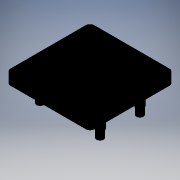
# Autodesk Inventor part: HFC5-2020-B
Saved by Autodesk Inventor 2017.3 (Build 213256000, 256)
## iProperties
Part Number: HFC5-2020-B
Material: Generic
Catalog Web Link: www.cadenas.de
Description: HFC5, HFCL5-Extrusion End Caps - HFS5 Series (Aluminum Extrusions 20, 25, 40 Square)
Vendor: MISUMI
Document SubType Name: Modeling
Designer: partserver
Manufacturer: MISUMI
Mass: 0.806307 g
Surface Area: 12.096 cm^2
Volume: 0.806307 cm^3
Density: 1 g/cm^3
Appearance: PSOLRGB-0-0-0
Category: PARTsolutions
Company: MISUMI
Title: HFC5-2020-B
Author: Cadenas PARTsolutions
Comments: Extrusion End Caps - HFS5 Series (Aluminum Extrusions 20, 25, 40 Square)
PSOL_IDENT_0: {$CADENAS_DATA\23d-libs\misumi\metric\38_al_extrusions_blackets\hfc5.prj},176 {VTYP=3D},{NB=HFC5-202
PSOL_IDENT_1: 0-B},{LINA=HFC5-2020-B},{NN=HFC5, HFCL5},{DATE=16.12.2019 05:49:00},{GEOMDATE=09.12.2019 01:53:00},{
PSOL_IDENT_2: VERSION=},{LINEID=10},{WBVAR=MAT,COLOR},{WBNUMERIC=}  {NB=HFC5-2020-B},{LINA=HFC5-2020-B},{KT=HFC5},
PSOL_IDENT_3: {PN=HFC5-2020-B},{TYPE=HFC5},{MAT=P},{MATALG='P','Polyamide','LDP','Low Density Polyethylene'},{NO=2
PSOL_IDENT_4: 020},{COLOR=B},{COL=0.00,0.00,0.00,0.00},{SHP3D=2020}
NB: HFC5-2020-B
NN: HFC5, HFCL5
NT: Extrusion End Caps - HFS5 Series (Aluminum Extrusions 20, 25, 40 Square)
NBSYN: $PN.
LINA: HFC5-2020-B
CATALOG: Misumi
PN: HFC5-2020-B
MAT: Polyamide
NO: 2020
COLOR: B (Black)
SUPPLIER: MISUMI
ARTICLENO: HFC5-2020-B
BOMINFO: HFC5-2020-B
CREATOR: CADENAS GmbH
Autodesk Inventor part; units mm, degrees
ref_plane "YZ Plane" through (0, 0, 0) normal (1, 0, 0) x (0, 1, 0)
ref_plane "XZ Plane" through (0, 0, 0) normal (0, 1, 0) x (-1, 0, 0)
ref_plane "XY Plane" through (0, 0, 0) normal (0, 0, 1) x (1, 0, 0)
sketch "Sketch_1" plane through (0, 0, 0) normal (0, 0, 1) x (1, 0, 0)
  arc A0 (-10, -9) -> (-9, -10) centre (-9, -9) ccw
  line L0 (-9, -10) -> (9, -10)
  arc A1 (9, -10) -> (10, -9) centre (9, -9) ccw
  line L1 (10, -9) -> (10, 9)
  arc A2 (10, 9) -> (9, 10) centre (9, 9) ccw
  line L2 (9, 10) -> (-9, 10)
  arc A3 (-9, 10) -> (-10, 9) centre (-9, 9) ccw
  line L3 (-10, 9) -> (-10, -9)
  constraints: 8 end point, 8 point on circle, 4 centre point
extrude "Extrusion1" add sketch "Sketch_1" against normal blind 2.5
sketch "Sketch_2" plane through (0, 0, 0) normal (0, 0, 1) x (1, 0, 0)
  arc A0 (-8, 6.3367) -> (-8, 3.1633) centre (-7.15, 4.75) ccw
  line L0 (-8, 3.1633) -> (-8, -3.1633)
  arc A1 (-8, -3.1633) -> (-8, -6.3367) centre (-7.15, -4.75) ccw
  line L1 (-8, -6.3367) -> (-8, -8)
  line L2 (-8, -8) -> (8, -8)
  line L3 (8, -8) -> (8, -6.3367)
  arc A2 (8, -6.3367) -> (8, -3.1633) centre (7.15, -4.75) ccw
  line L4 (8, -3.1633) -> (8, 3.1633)
  arc A3 (8, 3.1633) -> (8, 6.3367) centre (7.15, 4.75) ccw
  line L5 (8, 6.3367) -> (8, 8)
  line L6 (8, 8) -> (-8, 8)
  line L7 (-8, 8) -> (-8, 6.3367)
  constraints: 16 end point, 8 point on circle, 4 centre point
extrude "Extrusion2" cut sketch "Sketch_2" against normal blind 1
sketch "Sketch_3" plane through (0, 4.75, 0) normal (0, 1, 0) x (1, 0, 0)
  line L0 (-7.15, 1) -> (-7.15, -5.3)
  line L1 (-7.15, -5.3) -> (-8, -5.3)
  line L2 (-8, -5.3) -> (-8, -3.8)
  line L3 (-8, -3.8) -> (-8.15, -3.3)
  line L4 (-8.15, -3.3) -> (-8.15, 1)
  line L5 (-8.15, 1) -> (-7.15, 1)
  line L6 (-7.15, 1) -> (-7.15, -5.3)
  constraints: 14 end point
revolve "Revolution1" add sketch "Sketch_3" angle 360 about axis through (-7.15, 4.75, -1) along (0, 0, -1)
pattern_linear "Rectangular Pattern1" count 2 spacing 14.3 along (1, 0, 0) count 2 spacing 9.5 along (0, -1, 0) of "Revolution1"
ref_plane "Cap_to_Frame_XY" through (0, 0, 0) normal (0, 0, -1) x (1, 0, 0)
ref_plane "Cap_to_Frame_YZ" through (0, 0, 0) normal (1, 0, 0) x (0, -1, 0)
ref_plane "Cap_to_Frame_ZX" through (0, 0, 0) normal (0, -1, 0) x (0, 0, -1)
body "Solid1"
